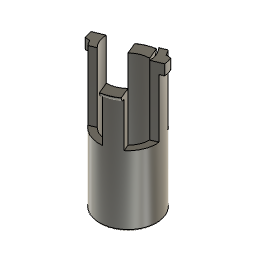
Cherry Pushbutton Insert (Autodesk Fusion 360 design; units mm, degrees)
Autodesk Fusion 360 part; units mm, degrees
sketch "Sketch1" plane through (0, 0, 0) normal (0, 0, 1) x (1, 0, 0)
  circle A0 centre (0, 0) radius 4.3625
  circle A1 centre (0, 0) radius 3.3274
  line L0 (0, 4.3624) -> (0, 0)
  line L1 (0, 0) -> (0, -4.3625)
  line L2 (-4.3625, 0) -> (0, 0)
  line L3 (4.3625, 0) -> (0, 0)
  line L4 (0, 0) -> (3.0847, 3.0847)
  line L5 (0, 0) -> (-3.0847, -3.0847)
  line L6 (-3.0847, 3.0847) -> (0, 0)
  line L7 (0, 0) -> (3.0847, -3.0847)
  line L8 (-2.7732, 3.3676) -> (-0.4203, 4.3422)
  line L9 (-0.4203, 4.3422) -> (2.7732, -3.3676)
  line L10 (2.7732, -3.3676) -> (0.4203, -4.3422)
  line L11 (0.4203, -4.3422) -> (-2.7732, 3.3676)
  line L12 (-3.3676, -2.7732) -> (-4.3422, -0.4203)
  line L13 (-4.3422, -0.4203) -> (3.3676, 2.7732)
  line L14 (3.3676, 2.7732) -> (4.3422, 0.4203)
  line L15 (4.3422, 0.4203) -> (-3.3676, -2.7732)
  point P0 (-2.3528, -2.3528)
  point P1 (-3.3274, 0)
  point P2 (0, -3.3274)
  point P3 (2.3528, -2.3528)
  point P4 (0, 3.3274)
  point P5 (-2.3528, 2.3528)
  dimension "d4" = 8.7249
  dimension "d5" = 6.6548
  dimension "d6" = 45
  constraint coincident A0.centre A1.centre
  constraint concentric A0 A1
  constraint parallel L0 L1
  constraint horizontal L3
  constraint parallel L2 L3
  constraint vertical L0
  constraint coincident A0 L4.end
  constraint coincident A0 L12.start
  constraint parallel L4 L5
  constraint coincident A0 L7.end
  constraint parallel L6 L7
  constraint perpendicular L5 L6
  constraint perpendicular L8 L9
  constraint parallel L8 L10
  constraint parallel L9 L11
  constraint perpendicular L12 L13
  constraint parallel L12 L14
  constraint parallel L13 L15
  constraint coincident L14.end L15.start
  constraint coincident A0 L3.start
  constraint coincident A0 L5.end
  constraint coincident A0 L12.end
  constraint coincident L12.end L13.start
  constraint coincident A0 L2.start
  constraint coincident L5 P0
  constraint coincident A1 P0
  constraint coincident L15 P0
  constraint coincident L2 P1
  constraint coincident A1 P1
  constraint coincident L13 P1
  constraint coincident A0 L13.end
  constraint coincident L10.end L11.start
  constraint coincident A0 L1.end
  constraint coincident A1 P2
  constraint coincident L1 P2
  constraint coincident L7 P3
  constraint coincident A1 P3
  constraint coincident A0 L6.start
  constraint coincident A0 L8.end
  constraint coincident A0 L0.start
  constraint coincident L0 P4
  constraint coincident A1 P4
  constraint coincident A1 P5
  constraint coincident L6 P5
  constraint coincident L11 P5
  constraint coincident L9 P4
  constraint coincident A0 L8.start
  constraint coincident A0 L9.end
  measures "d4" diameter of A0
  measures "d5" diameter of A1
  measures "d6" angle of L0 L6
extrude "Extrude1" add sketch "Sketch1" along normal blind 1.143 contours A1 L3 L4 L9 | L3 L9 L15 | A1 L9 L15 | A1 L1 L7 L15 | L7 L9 L15 | A1 L9 L13 | L4 L9 L13 | L3 L7 L9 L15 | L3 L4 L9 | L1 L11 L15 | A1 L11 L15 | L1 L7 L15 | A1 L0 L6 L13 | L0 L9 L13 | L0 L4 L9 L13 | L0 L6 L13 | L2 L5 L11 | L1 L5 L11 L15 | L2 L6 L11 L13 | A1 L2 L5 L11 | L5 L11 L15 | A1 L11 L13 | L6 L11 L13 | L2 L11 L13
extrude "Extrude2" add sketch "Sketch1" along normal blind 18.2372 contours A1 L9 L10 L11 | A0 L10 | A1 L8 L9 L11 | A0 L8
extrude "Extrude3" add sketch "Sketch1" along normal blind 21.2852 contours A0 L14 | A1 L13 L14 L15 | A1 L12 L13 L15 | A0 L12
extrude "Extrude4" add sketch "Sketch1" along normal blind 10.7156 contours A0 L3 L15 | A0 A1 L3 L7 | A0 L7 L9 | A0 L4 L13 | A0 A1 L0 L4 | A0 L1 L11 | A0 A1 L1 L5 | A0 L0 L9 | A0 L5 L15 | A0 A1 L2 L6 | A0 L6 L11 | A0 L2 L13
sketch "Sketch2" plane through (0, 0, 18.2372) normal (0, 0, 1) x (-1, 0, 0)
  arc A0 (0.4203, -4.3422) -> (2.7732, -3.3676) centre (0, 0) ccw
  line L0 (2.7732, -3.3676) -> (2.3528, -2.3528)
  arc A1 (0, -3.3274) -> (2.3528, -2.3528) centre (0, 0) ccw
  line L1 (0, -3.3274) -> (0.4203, -4.3422)
  arc A2 (-0.4203, 4.3422) -> (-2.7732, 3.3676) centre (0, 0) ccw
  line L2 (-2.7732, 3.3676) -> (-2.3528, 2.3528)
  arc A3 (-2.3528, 2.3528) -> (0, 3.3274) centre (0, 0) cw
  line L3 (0, 3.3274) -> (-0.4203, 4.3422)
  circle A4 centre (0, 0) radius 5.1435
  line L4 (2.7732, -3.3676) -> (0.4203, -4.3422)
  line L5 (0.4203, -4.3422) -> (0.7306, -5.0913)
  line L6 (0.7306, -5.0913) -> (3.0835, -4.1168)
  line L7 (3.0835, -4.1168) -> (2.7732, -3.3676)
  line L8 (-0.4203, 4.3422) -> (-2.7732, 3.3676)
  line L9 (-2.7732, 3.3676) -> (-3.0835, 4.1168)
  line L10 (-3.0835, 4.1168) -> (-0.7306, 5.0913)
  line L11 (-0.7306, 5.0913) -> (-0.4203, 4.3422)
  dimension "d18" = 10.287
  constraint concentric A0 A4
  constraint perpendicular L4 L5
  constraint parallel L4 L6
  constraint parallel L5 L7
  constraint coincident A0.start L1.end
  constraint perpendicular L1 L4
  constraint coincident A0.end L0.start
  constraint perpendicular L8 L9
  constraint parallel L8 L10
  constraint parallel L9 L11
  constraint coincident A2.end L2.start
  constraint perpendicular L2 L8
  constraint coincident A2.start L3.end
  constraint coincident A4 L5.end
  constraint coincident A4 L9.end
  measures "d18" diameter of A4
extrude "Extrude5" add sketch "Sketch2" against normal blind 0.762 contours A0 L5 L6 L7 | A4 L6 | A2 L9 L10 L11 | A4 L10
fillet "Fillet1" radius 0.75 2 edges at (1.9683, -4.752, 17.4752) (-1.9683, 4.752, 17.4752)
sketch "Sketch3" plane through (0, 0, 21.2852) normal (0, 0, 1) x (-1, 0, 0)
  arc A0 (-4.3422, -0.4203) -> (-3.3676, -2.7732) centre (0, 0) ccw
  line L0 (-3.3676, -2.7732) -> (-2.3528, -2.3528)
  arc A1 (-3.3274, 0) -> (-2.3528, -2.3528) centre (0, 0) ccw
  line L1 (-3.3274, 0) -> (-4.3422, -0.4203)
  arc A2 (4.3422, 0.4203) -> (3.3676, 2.7732) centre (0, 0) ccw
  line L2 (3.3676, 2.7732) -> (2.3528, 2.3528)
  arc A3 (2.3528, 2.3528) -> (3.3274, 0) centre (0, 0) cw
  line L3 (3.3274, 0) -> (4.3422, 0.4203)
  circle A4 centre (0, 0) radius 5.0038
  line L4 (4.3422, 0.4203) -> (3.3676, 2.7732)
  line L5 (3.3676, 2.7732) -> (3.9834, 3.0282)
  line L6 (3.9834, 3.0282) -> (4.958, 0.6754)
  line L7 (4.958, 0.6754) -> (4.3422, 0.4203)
  line L8 (-3.3676, -2.7732) -> (-4.3422, -0.4203)
  line L9 (-4.3422, -0.4203) -> (-4.958, -0.6754)
  line L10 (-4.958, -0.6754) -> (-3.9834, -3.0282)
  line L11 (-3.9834, -3.0282) -> (-3.3676, -2.7732)
  line L12 (-4.958, -0.6754) -> (-4.6283, -1.9019) construction
  line L13 (-3.3676, -2.7732) -> (-3.895, -1.9648) construction
  line L14 (-3.895, -1.9648) -> (-4.6283, -1.9019)
  line L15 (4.958, 0.6754) -> (4.6283, 1.9019) construction
  line L16 (3.3676, 2.7732) -> (3.895, 1.9648) construction
  line L17 (3.895, 1.9648) -> (4.6283, 1.9019)
  dimension "d26" = 10.0076
  dimension "d29" = 1.27
  dimension "d30" = 0.9652
  dimension "d35" = 1.27
  dimension "d36" = 0.9652
  constraint concentric A2 A4
  constraint perpendicular L4 L5
  constraint parallel L4 L6
  constraint parallel L5 L7
  constraint coincident A2.end L2.start
  constraint perpendicular L2 L4
  constraint coincident A2.start L3.end
  constraint perpendicular L8 L9
  constraint parallel L8 L10
  constraint parallel L9 L11
  constraint coincident A0.start L1.end
  constraint perpendicular L1 L8
  constraint coincident A0.end L0.start
  constraint coincident A4 L10.end
  constraint coincident A4 L6.end
  constraint coincident A4 L12.end
  constraint coincident A0 L13.end
  constraint coincident A4 L15.end
  constraint coincident A2 L16.end
  measures "d26" diameter of A4
  measures "d29" distance of L9.end L12.end
  measures "d30" distance of A0.end L13.end
  measures "d35" distance of L6.end L15.end
  measures "d36" distance of A2.end L16.end
extrude "Extrude6" add sketch "Sketch3" against normal blind 1.6002 contours A0 L9 L10 L14 | A4 L10 L14 | A4 L6 L17 | A2 L6 L7 L17 picked at (-4.6148, -1.7742) picked at (4.6148, 1.7742)
fillet "Fillet2" radius 0.254 1 edges at (-4.0672, -1.5775, 0)
equation "OutsideDiameter = 0.3435 in"
equation "InsideDiameter = 0.262 in"
equation "CoreHeight = ( 27 / 64 ) * 1 in"
equation "d4 = OutsideDiameter"
equation "d5 = InsideDiameter"
equation "ShortHeight = 0.718 in"
equation "LongHeight = 0.838 in"
equation "d11 = ShortHeight"
equation "d13 = LongHeight"
equation "d15 = CoreHeight"
equation "ShortFeetDiameter = 0.405 in"
equation "d18 = ShortFeetDiameter"
equation "d19 = -ShortFeetHeight"
equation "ShortFeetHeight = 0.03 in"
equation "LongFeetDiameter = 0.394 in"
equation "LongFeetHeight = 0.063 in"
equation "d26 = LongFeetDiameter"
equation "d27 = -LongFeetHeight"
equation "d29 = LongFootTabDistance"
equation "d30 = LongFootGapDistance"
equation "LongFootTabDistance = 0.05 in"
equation "LongFootGapDistance = 0.038 in"
equation "d35 = LongFootTabDistance"
equation "d36 = LongFootGapDistance"
